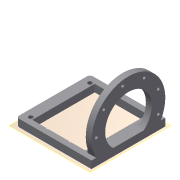
# Autodesk Inventor part: 30_Cube_LED_Array_v0
Saved by Autodesk Inventor 2019 (Build 230136000, 136)
## iProperties
Created: 2018-05-25
Part Number: 30_Cube_LED_Array_v0
Material: Generisch
Document SubType Name: Modeling
Designer: diederichbenedict
Density: 1 g/cm^3
Appearance: Vorgabe
Mass: 9.27173 g
Surface Area: 66.0193 cm^2
Volume: 9.27173 cm^3
Author: diederichbenedict
Autodesk Inventor part; units mm, degrees
ref_plane "YZ Plane" through (0, 0, 0) normal (1, 0, 0) x (0, 1, 0)
ref_plane "XZ Plane" through (0, 0, 0) normal (0, 1, 0) x (-1, 0, 0)
ref_plane "XY Plane" through (0, 0, 0) normal (0, 0, 1) x (1, 0, 0)
ref_plane "Arbeitsebene1" through (0, 0, 0) normal (0, 0, 1) x (1, 0, 0)
sketch "Skizze1" plane through (0, 0, 0) normal (0, 0, 1) x (1, 0, 0)
  arc A0 (13.4381, 5.6873) -> (13.3881, 5.2) centre (15.7881, 5.2) ccw construction
  line L0 (13.4381, 5.6873) -> (13.4381, 7.6) construction
  line L1 (13.4381, 7.6) -> (15.7881, 7.6) construction
  arc A1 (18.1881, 5.2) -> (15.7881, 7.6) centre (15.7881, 5.2) ccw projected
  line L2 (18.1881, 5.2) -> (18.1881, -5.2) construction
  arc A2 (15.7881, -7.6) -> (18.1881, -5.2) centre (15.7881, -5.2) ccw projected
  line L3 (15.7881, -7.6) -> (13.4381, -7.6) construction
  line L4 (13.4381, -7.6) -> (13.4381, -5.6873) construction
  arc A3 (13.3881, -5.2) -> (13.4381, -5.6873) centre (15.7881, -5.2) ccw construction
  line L5 (13.3881, -5.2) -> (13.3881, 5.2) construction
  arc A4 (14.5, 9) -> (11.5, 6) centre (14.5, 6) ccw construction
  line L6 (11.5, -6) -> (11.5, 6) construction
  arc A5 (11.5, -6) -> (14.5, -9) centre (14.5, -6) ccw construction
  line L7 (14.9, -9) -> (14.5, -9) construction
  arc A6 (17.9, -12) -> (14.9, -9) centre (14.9, -12) ccw projected
  line L8 (17.9, -12) -> (17.9, -21.066) projected
  line L9 (6.7383, -21.066) -> (-6.9383, -21.066) projected
  line L10 (-17.9, -21.066) -> (-17.9, 21.066) projected
  line L11 (-17.9, 21.066) -> (17.9, 21.066) projected
  line L12 (17.9, 21.066) -> (17.9, 12) projected
  arc A7 (14.9, 9) -> (17.9, 12) centre (14.9, 12) ccw projected
  line L13 (14.5, 9) -> (14.9, 9) construction
  circle A8 centre (-20, 20) radius 1.6 construction
  circle A9 centre (20, -20) radius 1.6 construction
  circle A10 centre (-20, -20) radius 1.6 construction
  circle A11 centre (20, 20) radius 1.6 construction
  arc A12 (-22.9, 24.9) -> (-24.9, 22.9) centre (-22.9, 22.9) ccw projected
  line L14 (-24.9, 22.9) -> (-24.9, -22.9) projected
  arc A13 (-24.9, -22.9) -> (-22.9, -24.9) centre (-22.9, -22.9) ccw projected
  line L15 (-22.9, -24.9) -> (22.9, -24.9) projected
  arc A14 (22.9, -24.9) -> (24.9, -22.9) centre (22.9, -22.9) ccw projected
  line L16 (24.9, -22.9) -> (24.9, 22.9) projected
  arc A15 (24.9, 22.9) -> (22.9, 24.9) centre (22.9, 22.9) ccw projected
  line L17 (22.9, 24.9) -> (-22.9, 24.9) projected
  arc A16 (6.7383, -21.066) -> (8.3017, -21.066) centre (7.52, -20.62) ccw projected
  arc A17 (-8.5017, -21.066) -> (-6.9383, -21.066) centre (-7.72, -20.62) ccw projected
  line L18 (-8.5017, -21.066) -> (-17.9, -21.066) projected
  line L19 (17.9, -21.066) -> (8.3017, -21.066) projected
  line L20 (17.9, -12) -> (17.9, 12)
  circle A18 centre (-20, 20) radius 1.4
  line L21 (-20, 20) -> (20, 20) construction
  line L22 (20, 20) -> (20, -20) construction
  line L23 (20, -20) -> (-20, -20) construction
  line L24 (-20, -20) -> (-20, 20) construction
  circle A19 centre (20, -20) radius 1.4
  circle A20 centre (20, 20) radius 1.4
  circle A21 centre (-20, -20) radius 1.4
  line L25 (25.9, -32.5) -> (25.9, 32.5) projected
  line L26 (22.9, -24.9) -> (25.9, -24.9)
  line L27 (22.9, 24.9) -> (25.9, 24.9)
  point P0 (0, 0)
  dimension "d7" = 2.8
  dimension "d8" = 40
  dimension "d9" = 40
  dimension "d10" = 2.8
  dimension "d11" = 2.8
  dimension "d12" = 2.8
  constraints: 14 end point, 4 centre point, 4 coincident, 3 perpendicular, 2 parallel, 2 point on line, 1 horizontal, 1 point on circle, 1 vertical
  measures "d7" diameter of A18
  measures "d8" distance of L22.end L23.end
  measures "d9" distance of L21.end L22.end
  measures "d10" diameter of A19
  measures "d11" diameter of A20
  measures "d12" diameter of A21
extrude "Extrusion1" add sketch "Skizze1" along normal blind 5
sketch "Sketch6" plane through (25.9, -24.9, 0) normal (1, 0, 0) x (0, 0, -1)
  circle A0 centre (-16.9, 25) radius 22.5 projected
  circle A1 centre (-16.9, 25) radius 15.75 projected
  line L0 (-5, 0) -> (-5, 49.8) projected
  line L1 (-5, 14.6824) -> (-5, 5.9045)
  line L2 (-5, 44.0955) -> (-5, 35.3176)
  arc A2 (-5, 46.8294) -> (-5, 3.1706) centre (-16.9, 25) ccw
  line L3 (-5, 46.8294) -> (-5, 35.3176)
  line L4 (-5, 14.6824) -> (-5, 3.1706)
  point P0 (0, 24.9)
  constraints: 8 end point, 6 point on circle, 6 point on line, 2 collinear, 1 centre point, 1 coincident
extrude "Extrusion3" add sketch "Sketch6" against normal blind 4 contours L0 A1 A0 | A0 L0 A2 picked at (-36.9413, 23.2431)
sketch "Sketch7" plane through (21.9, -24.9, 0) normal (-1, 0, 0) x (0, 0, 1)
  circle A0 centre (2.9774, 8.4941) radius 0.25 projected
  circle A1 centre (16.8445, 3.4065) radius 0.25 projected
  circle A2 centre (30.7375, 8.4227) radius 0.25 projected
  circle A3 centre (38.1558, 21.1956) radius 0.25 projected
  circle A4 centre (35.6283, 35.7487) radius 0.25 projected
  circle A5 centre (24.3376, 45.2723) radius 0.25 projected
  circle A6 centre (9.5668, 45.3103) radius 0.25 projected
  circle A7 centre (-1.7728, 35.8449) radius 0.25 projected
  circle A8 centre (-4.3751, 21.305) radius 0.25 projected
  line L0 (-2.665, 15.2234) -> (2.0334, 16.9335) projected
  line L1 (2.0334, 16.9335) -> (0.3233, 21.632) projected
  line L2 (0.3233, 21.632) -> (-4.3751, 19.9219) projected
  line L3 (-4.3751, 19.9219) -> (-2.665, 15.2234) projected
  line L4 (1.8587, 9.1214) -> (5.6889, 12.3353) projected
  line L5 (5.6889, 12.3353) -> (2.4749, 16.1656) projected
  line L6 (2.4749, 16.1656) -> (-1.3553, 12.9516) projected
  line L7 (-1.3553, 12.9516) -> (1.8587, 9.1214) projected
  line L8 (8.1966, 4.9346) -> (10.6966, 9.2647) projected
  line L9 (10.6966, 9.2647) -> (6.3664, 11.7647) projected
  line L10 (6.3664, 11.7647) -> (3.8664, 7.4346) projected
  line L11 (3.8664, 7.4346) -> (8.1966, 4.9346) projected
  line L12 (15.5842, 3.1679) -> (16.4525, 8.0919) projected
  line L13 (16.4525, 8.0919) -> (11.5284, 8.9602) projected
  line L14 (11.5284, 8.9602) -> (10.6602, 4.0361) projected
  line L15 (10.6602, 4.0361) -> (15.5842, 3.1679) projected
  line L16 (23.1306, 4.0345) -> (22.2623, 8.9586) projected
  line L17 (22.2623, 8.9586) -> (17.3383, 8.0903) projected
  line L18 (17.3383, 8.0903) -> (18.2066, 3.1663) projected
  line L19 (18.2066, 3.1663) -> (23.1306, 4.0345) projected
  line L20 (29.9255, 7.4299) -> (27.4255, 11.76) projected
  line L21 (27.4255, 11.76) -> (23.0953, 9.26) projected
  line L22 (23.0953, 9.26) -> (25.5953, 4.9299) projected
  line L23 (25.5953, 4.9299) -> (29.9255, 7.4299) projected
  line L24 (35.1493, 12.9445) -> (31.319, 16.1584) projected
  line L25 (31.319, 16.1584) -> (28.1051, 12.3282) projected
  line L26 (28.1051, 12.3282) -> (31.9353, 9.1142) projected
  line L27 (31.9353, 9.1142) -> (35.1493, 12.9445) projected
  line L28 (38.1719, 19.9131) -> (33.4735, 21.6232) projected
  line L29 (33.4735, 21.6232) -> (31.7634, 16.9247) projected
  line L30 (31.7634, 16.9247) -> (36.4618, 15.2146) projected
  line L31 (36.4618, 15.2146) -> (38.1719, 19.9131) projected
  line L32 (38.6289, 27.4953) -> (33.6289, 27.4953) projected
  line L33 (33.6289, 27.4953) -> (33.6289, 22.4953) projected
  line L34 (33.6289, 22.4953) -> (38.6289, 22.4953) projected
  line L35 (38.6289, 22.4953) -> (38.6289, 27.4953) projected
  line L36 (36.465, 34.7766) -> (31.7666, 33.0665) projected
  line L37 (31.7666, 33.0665) -> (33.4767, 28.368) projected
  line L38 (33.4767, 28.368) -> (38.1751, 30.0781) projected
  line L39 (38.1751, 30.0781) -> (36.465, 34.7766) projected
  line L40 (31.9413, 40.8786) -> (28.1111, 37.6647) projected
  line L41 (28.1111, 37.6647) -> (31.3251, 33.8344) projected
  line L42 (31.3251, 33.8344) -> (35.1553, 37.0484) projected
  line L43 (35.1553, 37.0484) -> (31.9413, 40.8786) projected
  line L44 (25.6034, 45.0654) -> (23.1034, 40.7353) projected
  line L45 (23.1034, 40.7353) -> (27.4336, 38.2353) projected
  line L46 (27.4336, 38.2353) -> (29.9336, 42.5654) projected
  line L47 (29.9336, 42.5654) -> (25.6034, 45.0654) projected
  line L48 (18.2158, 46.8321) -> (17.3475, 41.9081) projected
  line L49 (17.3475, 41.9081) -> (22.2716, 41.0398) projected
  line L50 (22.2716, 41.0398) -> (23.1398, 45.9639) projected
  line L51 (23.1398, 45.9639) -> (18.2158, 46.8321) projected
  line L52 (10.6694, 45.9655) -> (11.5377, 41.0414) projected
  line L53 (11.5377, 41.0414) -> (16.4617, 41.9097) projected
  line L54 (16.4617, 41.9097) -> (15.5934, 46.8337) projected
  line L55 (15.5934, 46.8337) -> (10.6694, 45.9655) projected
  line L56 (3.8745, 42.5701) -> (6.3745, 38.24) projected
  line L57 (6.3745, 38.24) -> (10.7047, 40.74) projected
  line L58 (10.7047, 40.74) -> (8.2047, 45.0701) projected
  line L59 (8.2047, 45.0701) -> (3.8745, 42.5701) projected
  line L60 (-1.3493, 37.0555) -> (2.481, 33.8416) projected
  line L61 (2.481, 33.8416) -> (5.6949, 37.6718) projected
  line L62 (5.6949, 37.6718) -> (1.8647, 40.8858) projected
  line L63 (1.8647, 40.8858) -> (-1.3493, 37.0555) projected
  line L64 (-4.3719, 30.0869) -> (0.3265, 28.3768) projected
  line L65 (0.3265, 28.3768) -> (2.0366, 33.0753) projected
  line L66 (2.0366, 33.0753) -> (-2.6618, 34.7854) projected
  line L67 (-2.6618, 34.7854) -> (-4.3719, 30.0869) projected
  line L68 (-4.8289, 22.5047) -> (0.1711, 22.5047) projected
  line L69 (0.1711, 22.5047) -> (0.1711, 27.5047) projected
  line L70 (0.1711, 27.5047) -> (-4.8289, 27.5047) projected
  line L71 (-4.8289, 27.5047) -> (-4.8289, 22.5047) projected
  circle A9 centre (16.9, 25) radius 15.75 projected
  circle A10 centre (16.9, 25) radius 22.5 projected
  point P0 (0, 24.9)
hole "Hole1" at (21.9, 20.4103, 9.5668) at (21.9, 20.3723, 24.3376) at (21.9, 10.8487, 35.6283) at (21.9, -3.7044, 38.1558) at (21.9, -16.4773, 30.7375) at (21.9, -21.4935, 16.8445) direction (1, 0, 0) diameter 2 end through all
fillet "Fillet2" radius 3.2 2 edges at (21.9, 16.1735, 5) (21.9, -15.9735, 5)
